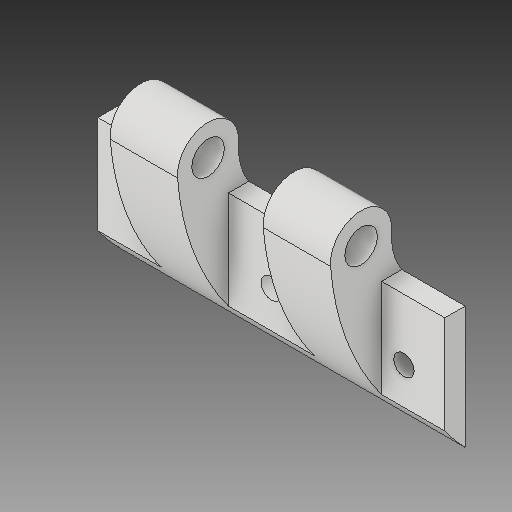
# Autodesk Inventor part: TC007b
Saved by Autodesk Inventor 2017 SP1 (Build 210196100, 196)
## iProperties
Created: 2018-01-07
Part Number: TC007b
Material: ABS Plastic
Document SubType Name: Modeling
Designer: Zach
Density: 1.06 g/cm^3
Appearance: CR White
Mass: 23.9702 g
Surface Area: 96.5634 cm^2
Volume: 22.6134 cm^3
Author: Zach
Autodesk Inventor part; units mm, degrees
ref_plane "YZ Plane" through (0, 0, 0) normal (1, 0, 0) x (0, 1, 0)
sketch "Sketch1" plane through (0, 0, 0) normal (0, 0, 1) x (1, 0, 0)
  line L0 (0, 0) -> (75, 0)
  line L1 (75, 0) -> (75, 30)
  line L2 (75, 30) -> (0, 30)
  line L3 (0, 30) -> (0, 0)
  point P0 (75, 15)
  point P1 (37.5, 30)
  dimension "d0" = 75
  dimension "d1" = 30
  constraints: 8 end point, 2 midpoint, 2 parallel, 1 horizontal, 1 perpendicular
  measures "d0" distance of L2.end L1.end
  measures "d1" distance of L1.end L0.end
extrude "Extrusion1" add sketch "Sketch1" along normal blind 5
ref_plane "Work Plane1" through (64.5, 0, 0) normal (1, 0, 0) x (0, 0, -1)
sketch "Sketch2" plane through (64.5, 0, 0) normal (1, 0, 0) x (0, 0, -1)
  circle A0 centre (-10, 40) radius 4
  circle A1 centre (-10, 40) radius 7.5 construction
  arc A2 (-17.4763, 39.4047) -> (0, 0) centre (47.3186, 44.564) ccw
  arc A3 (-2.5195, 39.4597) -> (-17.4763, 39.4047) centre (-10, 40) ccw
  arc A4 (-2.5195, 39.4597) -> (0, 30) centre (12.4415, 38.379) ccw
  line L0 (0, 30) -> (-5, 30) projected
  line L1 (0, 0) -> (0, 30) construction
  line L2 (0, 30) -> (0, 0)
  dimension "d8" = 8
  dimension "d9" = 15
  dimension "d13" = 65
  dimension "d26" = 15
  dimension "d27" = 10
  dimension "d28" = 10
  constraints: 8 point on circle, 5 centre point, 3 tangent, 2 coincident, 2 end point, 1 vertical
  measures "d8" diameter of A0
  measures "d9" diameter of A1
  measures "d13" radius of A2
  measures "d26" radius of A4
  measures "d27" horizontal distance of L0.start A0.centre
  measures "d28" horizontal distance of A0.centre L0.start
extrude "Extrusion2" add sketch "Sketch2" against normal blind 16.5
ref_plane "Work Plane2" through (10.5, 0, 0) normal (-1, 0, 0) x (0, 0, 1)
sketch "Sketch3" plane through (10.5, 0, 0) normal (-1, 0, 0) x (0, 0, 1)
  circle A0 centre (10, 40) radius 4 projected
  line L0 (5, 5.9924) -> (5, 30) projected
  arc A1 (5, 5.9924) -> (17.4763, 39.4047) centre (-47.3186, 44.564) ccw projected
  arc A2 (17.4763, 39.4047) -> (2.5195, 39.4597) centre (10, 40) ccw projected
  line L1 (5, 30) -> (0, 30) projected
  arc A3 (0, 30) -> (2.5195, 39.4597) centre (-12.4415, 38.379) ccw projected
  point P0 (0, 0)
extrude "Extrusion3" add sketch "Sketch3" against normal blind 16.5
sketch "Sketch7" plane through (0, 0, 5) normal (0, 0, 1) x (1, 0, 0)
  line L0 (5, 15) -> (70, 15) construction
  line L1 (0, 0) -> (75, 0) projected
  circle A0 centre (5, 15) radius 2.5
  circle A1 centre (37.5, 15) radius 2.5
  circle A2 centre (70, 15) radius 2.5
  line L2 (0, 30) -> (0, 0) projected
  point P0 (37.5, 0)
  point P1 (0, 15)
  dimension "d29" = 65
  dimension "d30" = 5
  dimension "d31" = 5
  dimension "d32" = 5
  constraints: 3 centre point, 3 coincident, 3 midpoint, 2 end point, 1 horizontal, 1 horizontal alignment, 1 vertical alignment
  measures "d29" distance of L0.start L0.end
  measures "d30" diameter of A0
  measures "d31" diameter of A1
  measures "d32" diameter of A2
extrude "Extrusion6" cut sketch "Sketch7" against normal through all
sketch "Sketch9" plane through (0, 0, 5) normal (0, 0, 1) x (1, 0, 0)
  line L0 (10.5, 30) -> (0, 30) projected
  line L1 (0, 30) -> (-5, 30)
  line L2 (-5, 30) -> (-5, 0)
  line L3 (-5, 0) -> (0, 0)
  line L4 (0, 0) -> (0, 30)
  line L5 (0, 0) -> (75, 0) projected
  line L6 (75, 0) -> (80, 0)
  line L7 (80, 0) -> (80, 30)
  line L8 (80, 30) -> (75, 30)
  line L9 (75, 30) -> (75, 0)
  point P0 (-2.5, 0)
  dimension "d37" = 5
  dimension "d38" = 5
  constraints: 16 end point, 4 parallel, 2 horizontal, 2 perpendicular, 1 horizontal alignment, 1 midpoint, 1 point on line
  measures "d37" distance of L3.end L2.end
  measures "d38" distance of L8.end L7.end
extrude "Extrusion8" add sketch "Sketch9" against normal blind 5
sketch "Sketch8" plane through (10.5, 0, 0) normal (-1, 0, 0) x (0, 0, 1)
  arc A0 (5, 5.9924) -> (17.4763, 39.4047) centre (-47.3186, 44.564) ccw construction
  arc A1 (0, 0) -> (17.4763, 39.4047) centre (-47.3186, 44.564) ccw construction
  line L0 (5, 0) -> (5, 30) projected
  line L1 (5, 5.9924) -> (5, 0)
  line L2 (5, 0) -> (0, 0)
  arc A2 (0, 0) -> (5, 5.9924) centre (-47.3186, 44.564) ccw
  constraints: 4 end point, 4 point on circle, 2 centre point, 2 concentric, 1 collinear, 1 perpendicular
extrude "Extrusion7" cut sketch "Sketch8" along normal through all both and the other way through all
body "Solid1"
